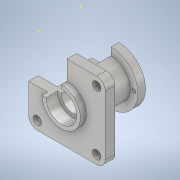
# Autodesk Inventor part: pieza 23.xx.2
Saved by Autodesk Inventor 2020 (Build 240168000, 168)
## iProperties
Created: 2020-04-21
Part Number: pieza 23.xx.2
Material: Titanio
Document SubType Name: Modeling
Designer: davidesteban
Density: 4.51 g/cm^3
Appearance: Aluminio - Oscuro
Author: Luis Gallardo
Autodesk Inventor part; units mm, degrees
ref_plane "YZ Plane" through (0, 0, 0) normal (1, 0, 0) x (0, 1, 0)
ref_plane "XZ Plane" through (0, 0, 0) normal (0, 1, 0) x (-1, 0, 0)
ref_plane "XY Plane" through (0, 0, 0) normal (0, 0, 1) x (1, 0, 0)
ref_plane "Plano de trabajo4" through (0, 0, -10) normal (0, 0, -1) x (-1, 0, 0)
sketch "Boceto10" plane through (0, 0, -10) normal (0, 0, -1) x (-1, 0, 0)
  arc A0 (-40, -20) -> (-20, -40) centre (-40, -40) ccw projected
  line L0 (0, 0) -> (-80, 0)
  line L1 (-80, 0) -> (-80, -80)
  line L2 (-80, -80) -> (0, -80)
  line L3 (0, -80) -> (0, 0)
  dimension "d50" = 80
  dimension "d51" = 80
  constraints: 8 end point, 2 parallel, 1 horizontal, 1 perpendicular
  measures "d50" distance of L2.end L1.end
  measures "d51" distance of L1.end L0.end
extrude "Extrusión4" add sketch "Boceto10" along normal blind 10
sketch "Boceto11" plane through (0, 0, -20) normal (0, 0, -1) x (-1, 0, 0)
  arc A0 (-40, -20) -> (-20, -40) centre (-40, -40) ccw projected
  circle A1 centre (-40, -40) radius 20
  point P0 (0, 0)
  dimension "d54" = 40
  constraints: 1 centre point, 1 coincident
  measures "d54" diameter of A1
extrude "Extrusión5" add sketch "Boceto11" along normal blind 36
sketch "Boceto12" plane through (40, -40, -56) normal (0, 0, -1) x (-1, 0, 0)
  circle A0 centre (0, 0) radius 28
  point P0 (40, 40)
  dimension "d57" = 56
  constraints: 1 centre point
  measures "d57" diameter of A0
extrude "Extrusión6" add sketch "Boceto12" along normal blind 8
sketch "Boceto13" plane through (0, 0, -10) normal (0, 0, -1) x (-1, 0, 0)
  circle A0 centre (-40, -40) radius 20 projected
  circle A1 centre (-40, -40) radius 20
  circle A2 centre (-40, -40) radius 16
  point P0 (0, 0)
  dimension "d60" = 40
  dimension "d61" = 32
  constraints: 2 centre point, 2 coincident
  measures "d60" diameter of A1
  measures "d61" diameter of A2
extrude "Extrusión7" add sketch "Boceto13" against normal blind 6
sketch "Boceto14" plane through (0, 0, -10) normal (0, 0, -1) x (-1, 0, 0)
  circle A0 centre (-40, -40) radius 20 projected
  circle A1 centre (-40, -40) radius 16
  point P0 (0, 0)
  dimension "d64" = 32
  constraints: 1 centre point, 1 coincident
  measures "d64" diameter of A1
extrude "Extrusión8" cut sketch "Boceto14" along normal blind 6 contours A1
ref_plane "Plano de trabajo5" through (0, -40, -10) normal (0, 1, 0) x (1, 0, 0)
sketch "Boceto15" plane through (0, -40, -10) normal (0, 1, 0) x (1, 0, 0)
  line L0 (20, 10) -> (20, 46) projected
  line L1 (40, 68) -> (40, -62)
  line L2 (56, 6) -> (24, 6) projected
  line L3 (20, 6) -> (24, 6)
  line L4 (20, 10) -> (20, 42)
  line L5 (60, 10) -> (60, 46) projected
  line L6 (56, 6) -> (60, 6)
  line L7 (60, 6) -> (60, 38)
  line L8 (20, 42) -> (67, 42)
  line L9 (24, 6) -> (60.0219, 6) construction
  line L10 (24, 6) -> (28, 6)
  line L11 (56, 6) -> (52, 6)
  line L12 (28, 6) -> (29.1175, 38)
  line L13 (28, 6) -> (60.0195, 6) construction
  point P0 (0, -10)
  dimension "d68" = 4
  dimension "d69" = 32
  dimension "d70" = 32
  dimension "d75" = 4
  dimension "d76" = 4
  dimension "d77" = 88
  constraints: 22 end point, 4 point on line, 3 horizontal, 1 collinear, 1 equal length, 1 perpendicular, 1 vertical
  measures "d68" distance of L3.start L2.end
  measures "d69" distance of L0.start L4.end
  measures "d70" distance of L6.end L7.end
  measures "d75" distance of L2.end L10.end
  measures "d76" distance of L2.start L11.end
  measures "d77" angle of L13 L12
revolve "Revolución2" cut sketch "Boceto15" angle 360 about axis through (40, -40, -78) along (0, 0, 1) fills toward (28.6087, 21.9983) open curves L12
sketch "Boceto17" plane through (0, 0, -20) normal (0, 0, -1) x (-1, 0, 0)
  point P0 (0, 0)
sketch "Boceto18" plane through (40, -40, -64) normal (0, 0, -1) x (-1, 0, 0)
  circle A0 centre (0, 0) radius 15
  point P0 (40, 40)
  dimension "d80" = 30
  constraints: 1 centre point
  measures "d80" diameter of A0
extrude "Extrusión9" cut sketch "Boceto18" against normal blind 16
sketch "Boceto19" plane through (0, 0, -20) normal (0, 0, -1) x (-1, 0, 0)
  point P0 (0, 0)
sketch "Boceto20" plane through (0, 0, -10) normal (0, 0, -1) x (-1, 0, 0)
  line L0 (0, 0) -> (-80, 0) projected
  line L1 (0, 0) -> (-40, 0)
  line L2 (-40, 0) -> (-40, -40)
  line L3 (-40, -40) -> (0, -40)
  line L4 (0, -40) -> (0, 0)
  dimension "d83" = 40
  dimension "d84" = 40
  constraints: 8 end point, 2 parallel, 1 horizontal, 1 perpendicular
  measures "d83" distance of L3.end L2.end
  measures "d84" distance of L2.end L1.end
extrude "Extrusión10" cut sketch "Boceto20" against normal blind 6
sketch "Boceto21" plane through (0, 0, -10) normal (0, 0, -1) x (-1, 0, 0)
  circle A0 centre (-40, -40) radius 20 projected
  line L0 (0, 0) -> (-40, 0)
  line L1 (-40, 0) -> (-40, -40)
  line L2 (-40, -40) -> (0, -40)
  line L3 (0, -40) -> (0, 0)
  dimension "d87" = 40
  dimension "d88" = 40
  constraints: 8 end point, 2 parallel, 1 horizontal, 1 perpendicular
  measures "d87" distance of L2.end L1.end
  measures "d88" distance of L1.end L0.end
extrude "Extrusión11" cut sketch "Boceto21" along normal blind 55 contours L2 L1 A0 | A0 L1 L0 L3 L2 picked at (-27.494, -35.624)
fillet "Empalme7" radius 9 3 edges at (0, -80, -15) (80, -80, -15) (80, 0, -15)
sketch "Boceto22" plane through (0, 0, -10) normal (0, 0, -1) x (-1, 0, 0)
  arc A0 (-71, 0) -> (-80, -9) centre (-71, -9) ccw projected
  line L0 (-80, -9) -> (-80, -71) projected
  arc A1 (-80, -71) -> (-71, -80) centre (-71, -71) ccw projected
  line L1 (-71, -80) -> (-9, -80) projected
  arc A2 (-9, -80) -> (0, -71) centre (-9, -71) ccw projected
  line L2 (0, -71) -> (0, -40) projected
  line L3 (0, -40) -> (-20, -40) projected
  arc A3 (-40, -20) -> (-20, -40) centre (-40, -40) ccw projected
  line L4 (-40, -20) -> (-40, 0) projected
  line L5 (-40, 0) -> (-71, 0) projected
  circle A4 centre (-71, -71) radius 4.5
  circle A5 centre (-9, -71) radius 4.5
  circle A6 centre (-71, -9) radius 4.5
  point P0 (0, 0)
  dimension "d92" = 9
  dimension "d93" = 9
  dimension "d94" = 9
  constraints: 3 centre point, 3 coincident
  measures "d92" diameter of A4
  measures "d93" diameter of A5
  measures "d94" diameter of A6
extrude "Extrusión12" cut sketch "Boceto22" along normal blind 12 contours A4 | A5 | A6
ref_plane "Plano de trabajo6" through (40, -40, -64) normal (0, 0, -1) x (-1, 0, 0)
sketch "Boceto23" plane through (40, -40, -64) normal (0, 0, -1) x (-1, 0, 0)
  point P0 (40, 40)
sketch "Boceto24" plane through (40, -40, -64) normal (0, 0, -1) x (-1, 0, 0)
  line L0 (0, 0) -> (12, -20.7846)
  line L1 (0, 0) -> (24, 0) construction
  line L2 (0, 0) -> (-24, 0)
  circle A0 centre (12, -20.7846) radius 2
  circle A1 centre (-24, 0) radius 2
  point P0 (40, 40)
  dimension "d98" = 24
  dimension "d99" = 60
  dimension "d100" = 24
  dimension "d101" = 4
  dimension "d102" = 4
  constraints: 6 end point, 2 centre point, 2 coincident, 2 horizontal, 1 equal length
  measures "d98" distance of L0.start L0.end
  measures "d99" angle of L0 L1
  measures "d100" distance of L0.start L2.end
  measures "d101" diameter of A0
  measures "d102" diameter of A1
extrude "Extrusión13" cut sketch "Boceto24" against normal blind 9
